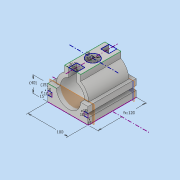
# Autodesk Inventor part: lw_3_ползунок
Saved by Autodesk Inventor 2019 (Build 230136000, 136)
## iProperties
Created: 2021-02-21
Part Number: lw_3_ползунок
Material: Типовые
Document SubType Name: ЛистМат
Designer: Kurbatova
Density: 1 g/cm^3
Appearance: По умолчанию
Sheet Metal Rule: По умолчанию
Author: Kurbatova
Autodesk Inventor part; units mm, degrees
ref_plane "YZ Plane" through (0, 0, 0) normal (1, 0, 0) x (0, 1, 0)
ref_plane "XZ Plane" through (0, 0, 0) normal (0, 1, 0) x (-1, 0, 0)
ref_plane "XY Plane" through (0, 0, 0) normal (0, 0, 1) x (1, 0, 0)
sketch "bottom" plane through (0, 0, 0) normal (0, 1, 0) x (-1, 0, 0)
  line L0 (53.8137, 54.0949) -> (-46.1863, 54.0949)
  line L1 (-46.1863, 54.0949) -> (-46.1863, -65.9051)
  line L2 (-46.1863, -65.9051) -> (53.8137, -65.9051)
  line L3 (53.8137, -65.9051) -> (53.8137, 54.0949)
  line L4 (102.7933, -5.9051) -> (-137.2052, -5.9051)
  point P0 (0, 0)
  point P1 (53.8137, -5.9051)
  dimension "d0" = 120
  dimension "d1" = 100
  constraints: 10 end point, 2 horizontal, 2 parallel, 1 midpoint, 1 perpendicular, 1 point on line
  measures "d0" distance between parallel lines of L2 L0
  measures "d1" distance between parallel lines of L1 L3
extrude "Выдавливание1" add sketch "bottom" along normal blind 40
sketch "tube" plane through (-53.8137, 0, 54.0949) normal (0, 0, 1) x (1, 0, 0)
  circle A0 centre (51.5912, 40) radius 30
  line L0 (51.5912, 113.4013) -> (51.5912, -34.7388)
  line L1 (0, 40) -> (100, 40) projected
  point P0 (53.8137, 0)
  dimension "d6" = 60
  constraints: 2 end point, 2 point on line, 1 centre point, 1 vertical
  measures "d6" diameter of A0
extrude "Углубление 1" cut sketch "tube" against normal blind 120
sketch "paz1" plane through (-53.8137, 0, 54.0949) normal (0, 0, 1) x (1, 0, 0)
  line L0 (0, 0) -> (100, 0) projected
  line L1 (-0.0635, 15) -> (9.9365, 15)
  line L2 (9.9365, 15) -> (9.9365, 25)
  line L3 (9.9365, 25) -> (-0.0635, 25)
  line L4 (-0.0635, 25) -> (-0.0635, 15)
  line L5 (0, 40) -> (21.5912, 40) projected
  line L6 (89.6996, 15) -> (99.6996, 15)
  line L7 (99.6996, 15) -> (99.6996, 25)
  line L8 (99.6996, 25) -> (89.6996, 25)
  line L9 (89.6996, 25) -> (89.6996, 15)
  point P0 (53.8137, 0)
  dimension "d11" = 10
  dimension "d12" = 10
  dimension "d13" = 15
  dimension "d14" = 15
  dimension "d15" = 40
  dimension "d16" = 10
  dimension "d17" = 10
  dimension "d18" = 15
  constraints: 18 end point, 6 perpendicular, 2 horizontal
  measures "d11" distance between parallel lines of L1 L3
  measures "d12" distance between parallel lines of L2 L4
  measures "d13" distance between parallel lines of L0 L1
  measures "d14" distance between parallel lines of L3 L5
  measures "d15" distance between parallel lines of L0 L5
  measures "d16" distance between parallel lines of L6 L8
  measures "d17" distance between parallel lines of L7 L9
  measures "d18" distance between parallel lines of L0 L6
extrude "Паз 1" cut sketch "paz1" against normal up to next contours L4 L3 L2 L1
sketch "paz2" plane through (-53.8137, 0, 54.0949) normal (0, 0, 1) x (1, 0, 0)
  line L0 (0, 0) -> (100, 0)
  line L1 (0, 15) -> (10, 15)
  line L2 (10, 15) -> (10, 25)
  line L3 (10, 25) -> (0, 25)
  line L4 (0, 25) -> (0, 15)
  line L5 (0, 40) -> (21.5912, 40)
  line L6 (50, 55.3447) -> (50, -18.8311)
  line L7 (100, 15) -> (90, 15)
  line L8 (90, 15) -> (90, 25)
  line L9 (90, 25) -> (100, 25)
  line L10 (100, 25) -> (100, 15)
  line L11 (-10.5586, 20) -> (107.965, 20)
  line L12 (100, 0) -> (100, 40) projected
  arc A0 (21.5912, 40) -> (81.5912, 40) centre (51.5912, 40) ccw projected
  line L13 (81.5912, 40) -> (100, 40)
  line L14 (100, 25) -> (100, 40)
  line L15 (100, 15) -> (100, 0)
  line L16 (0, 25) -> (0, 40) projected
  line L17 (0, 40) -> (0, 25)
  line L18 (0, 0) -> (100, 0) projected
  line L19 (0, 15) -> (0, 0)
  point P0 (53.8137, 0)
  point P1 (53.8137, 0)
  point P2 (50, 0)
  point P3 (100, 20)
  point P4 (100, 15)
  dimension "d21" = 10
  dimension "d22" = 10
  dimension "d23" = 15
  dimension "d24" = 15
  dimension "d25" = 40
  constraints: 36 end point, 4 symmetric about line, 3 horizontal, 3 midpoint, 3 perpendicular, 3 point on line, 3 vertical, 2 collinear
  measures "d21" distance between parallel lines of L1 L3
  measures "d22" distance between parallel lines of L2 L4
  measures "d23" distance between parallel lines of L0 L1
  measures "d24" distance between parallel lines of L3 L5
  measures "d25" distance between parallel lines of L0 L5
ref_plane "фронт1" through (-53.8137, 0, 44.0949) normal (0, 0, 1) x (1, 0, 0)
ref_plane "фронт2" through (46.1863, 0, -55.9051) normal (0, 0, -1) x (-1, 0, 0)
sketch "front_arc" plane through (-53.8137, 0, 44.0949) normal (0, 0, 1) x (1, 0, 0)
  arc A0 (21.5912, 40) -> (81.5912, 40) centre (51.5912, 40) ccw projected
  arc A1 (81.5912, 40) -> (21.5912, 40) centre (51.5912, 40) ccw
  line L0 (0, 40) -> (21.5912, 40) projected
  line L1 (81.5912, 40) -> (100, 40) projected
  line L2 (11.5912, 40) -> (21.5912, 40)
  line L3 (81.5912, 40) -> (91.5912, 40)
  line L4 (31.5912, 90) -> (31.5912, 74.641)
  line L5 (31.5912, 90) -> (51.5912, 90)
  line L6 (51.5912, 105.7627) -> (51.5912, 37.5467)
  line L7 (71.5912, 90) -> (71.5912, 74.641)
  line L8 (71.5912, 90) -> (51.5912, 90)
  arc A2 (91.5912, 40) -> (71.5912, 74.641) centre (51.5912, 40) ccw
  arc A3 (31.5912, 74.641) -> (11.5912, 40) centre (51.5912, 40) ccw
  point P0 (53.8137, 0)
  point P1 (31.5912, 40)
  point P2 (31.5912, 62.3607)
  point P3 (71.5912, 62.3607)
  dimension "d75" = 50
  dimension "d76" = 20
  dimension "d77" = 20
  constraints: 16 end point, 8 point on circle, 3 centre point, 2 coincident, 2 horizontal, 2 point on line, 2 symmetric about line, 2 vertical, 1 collinear, 1 concentric, 1 horizontal alignment
  measures "d75" distance of L4.start point (31.591, 40)
  measures "d76" distance from line of L4 A0.centre
  measures "d77" distance of L4.start L5.end
extrude "Выдавливание9" add sketch "front_arc" against normal blind 100 contours L0 A3 L4 L5 L6 A1 | A1 L6 L8 L7 A2 L1
sketch "top" plane through (-22.2225, 90, 44.0949) normal (0, 1, 0) x (1, 0, 0)
  line L0 (40, 0) -> (0, 0) projected
  line L1 (40, 0) -> (40, 100) projected
  line L2 (0, 100) -> (40, 100) projected
  line L3 (0, 0) -> (0, 100) projected
  line L4 (10, 0) -> (30, 0)
  line L5 (-37.6485, 50) -> (83.4602, 50)
  circle A0 centre (20, 50) radius 15
  line L6 (0, 100) -> (40, 100) projected
  line L7 (10, 20) -> (10, 0)
  line L8 (40, 0) -> (0, 0) projected
  line L9 (10, 20) -> (30, 20)
  line L10 (30, 20) -> (30, 0)
  line L11 (10, 100) -> (30, 100)
  line L12 (10, 80) -> (10, 100)
  line L13 (10, 80) -> (30, 80)
  line L14 (30, 80) -> (30, 100)
  line L15 (20, -16.8031) -> (20, 112.4511)
  point P0 (22.2225, 44.0949)
  point P1 (20, 0)
  point P2 (20, 100)
  point P3 (20, 100)
  dimension "d81" = 30
  dimension "d83" = 20
  dimension "d84" = 20
  dimension "d87" = 20
  constraints: 20 end point, 5 symmetric about line, 4 midpoint, 3 horizontal, 2 perpendicular, 1 centre point, 1 point on line, 1 vertical
  measures "d81" diameter of A0
  measures "d83" distance of L4.start L4.end
  measures "d84" distance of L7.start L4.start
  measures "d87" distance from line of A0.centre L3
extrude "Выдавливание10" cut sketch "top" against normal blind 30 contours L0 L15 L9 L10 | L0 L7 L9 L15 | L14 L13 L15 L2 | L15 L13 L12 L2
extrude "Выдавливание11" cut sketch "top" against normal blind 25 contours A0 L15 L5 | L5 L15 A0 | L15 A0 L5 | L5 A0 L15
extrude "Выдавливание12" cut sketch "paz2" against normal blind 120 contours L7 L8 L11 L10 | L11 L8 L9 L10
equation "\"Радиус_гибки\" = Толщина"
equation "\"Ширина_просечки\" = Толщина"
equation "\"Глубина_просечки\" = 0.5 * Толщина"
equation "\"Размер_просечки\" = 4 * Толщина"
equation "\"Мин_остаток\" = 2 * Толщина"
equation "\"Радиус_перехода\" = Радиус_гибки"
equation "\"Радиус_Якоби\" = Толщина"
equation "\"Размер_зазора\" = Толщина"
equation "\"Толщина\" = 0.5"
